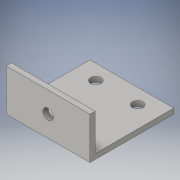
# Autodesk Inventor part: improved transmission bracket
Saved by Autodesk Inventor 2016 SP2 (Build 200236200, 236)
## iProperties
Created: 2018-01-20
Part Number: improved transmission bracket
Material: Generic
Document SubType Name: Modeling
Designer: CAD
Density: 1 g/cm^3
Appearance: Default
Author: CAD
Autodesk Inventor part; units mm, degrees
ref_plane "YZ Plane" through (0, 0, 0) normal (1, 0, 0) x (0, 1, 0)
ref_plane "XZ Plane" through (0, 0, 0) normal (0, 1, 0) x (-1, 0, 0)
ref_plane "XY Plane" through (0, 0, 0) normal (0, 0, 1) x (1, 0, 0)
sketch "Sketch1" plane through (0, 0, 0) normal (0, 1, 0) x (-1, 0, 0)
  line L0 (0, 0) -> (50.8, 0)
  line L1 (50.8, 0) -> (50.8, -50.8)
  line L2 (50.8, -50.8) -> (0, -50.8)
  line L3 (0, -50.8) -> (0, 0)
  dimension "d0" = 50.8
  dimension "d1" = 50.8
  constraints: 8 end point, 2 parallel, 1 horizontal, 1 perpendicular
  measures "d0" distance of L1.end L2.end
  measures "d1" distance of L0.end L1.end
extrude "Extrusion1" add sketch "Sketch1" along normal blind 3.175
sketch "Sketch2" plane through (0, 3.175, 0) normal (0, 1, 0) x (1, 0, 0)
  line L0 (-50.8, 0) -> (0, 0) projected
  line L1 (0, 0) -> (0, 50.8) projected
  line L2 (-50.8, 0) -> (0, 0)
  line L3 (0, 0) -> (0, 3.175)
  line L4 (0, 3.175) -> (-50.8, 3.175)
  line L5 (-50.8, 3.175) -> (-50.8, 0)
  dimension "d4" = 3.175
  constraints: 8 end point, 2 parallel, 1 horizontal, 1 perpendicular, 1 point on line
  measures "d4" distance between parallel lines of L0 L4
extrude "Extrusion2" add sketch "Sketch2" along normal blind 22.225
sketch "Sketch3" plane through (0, 3.175, 0) normal (0, 1, 0) x (1, 0, 0)
  line L0 (0, 3.175) -> (0, 50.8) projected
  line L1 (-50.8, 50.8) -> (-50.8, 3.175) projected
  line L2 (0, 50.8) -> (-50.8, 50.8) projected
  point P0 (0, 0)
  point P1 (-12.7, 41.656)
  point P2 (-38.1, 41.656)
  dimension "d9" = 9.144
  dimension "d10" = 9.144
  dimension "d18" = 25.4
  dimension "d19" = 12.7
  dimension "d20" = 12.7
  dimension "d21" = 50.8
  measures "d9" distance from line of L2 point (-12.7, 41.656)
  measures "d10" distance from line of L2 point (-38.1, 41.656)
  measures "d18" distance of point (-38.1, 41.656) point (-12.7, 41.656)
  measures "d19" distance from line of L0 point (-12.7, 41.656)
  measures "d20" distance from line of L1 point (-38.1, 41.656)
  measures "d21" distance of L0.end L1.start
hole "Hole1" at (-12.7, 3.175, -41.656) at (-38.1, 3.175, -41.656) direction (0, -1, 0) diameter 6.35 depth 25.4 tip angle 118
sketch "Sketch5" plane through (-50.8, 0, 0) normal (0, 0, 1) x (1, 0, 0)
  line L0 (0, 25.4) -> (50.8, 25.4) projected
  line L1 (50.8, 0) -> (50.8, 25.4) projected
  point P0 (25.4, 12.7)
  dimension "d23" = 12.7
  dimension "d24" = 25.4
  measures "d23" distance from line of L0 point (25.4, 12.7)
  measures "d24" distance from line of L1 point (25.4, 12.7)
hole "Hole2" at (-25.4, 12.7, 0) direction (0, 0, -1) diameter 6.35 end through all
equation "\"d10\" = d9"
equation "\"d19\" = -0.5 * d18 + 0.5 * d21"
body "Solid1"
